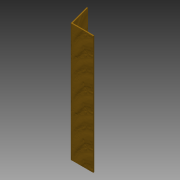
# Autodesk Inventor part: scharnierband
Saved by Autodesk Inventor 2017 (Build 210142000, 142)
## iProperties
Created: 2018-10-12
Part Number: scharnierband
Material: Brass, Soft Yellow, Welded
Document SubType Name: Modeling
Designer: ari
Density: 8.5 g/cm^3
Appearance: Weld - Brass
Author: ari
Autodesk Inventor part; units mm, degrees
ref_plane "YZ Plane" through (0, 0, 0) normal (1, 0, 0) x (0, 1, 0)
ref_plane "XZ Plane" through (0, 0, 0) normal (0, 1, 0) x (-1, 0, 0)
ref_plane "XY Plane" through (0, 0, 0) normal (0, 0, 1) x (1, 0, 0)
sketch "Sketch1" plane through (0, 0, 0) normal (0, 0, 1) x (1, 0, 0)
  line L0 (0, 0) -> (20, 0)
  line L1 (20, 0) -> (20, -1)
  line L2 (20, -1) -> (0, -1)
  line L3 (0, -1) -> (0, 0)
  line L4 (0, 0) -> (-5.1595, 19.323)
  line L5 (-5.1595, 19.323) -> (-6.1257, 19.0651)
  line L6 (-6.1257, 19.0651) -> (-0.9662, -0.258)
  line L7 (-0.9662, -0.258) -> (0, 0)
  circle A0 centre (-0.384, -0.5) radius 0.6304
  dimension "d0" = 20
  dimension "d1" = 1
  dimension "d2" = 104.95
  constraints: 16 end point, 4 parallel, 3 point on circle, 2 equal length, 2 perpendicular, 1 centre point, 1 horizontal
  measures "d0" distance of L1.end L2.end
  measures "d1" distance of L0.end L1.end
  measures "d2" angle of L4 L0
extrude "Extrusion1" add sketch "Sketch1" along normal blind 70 and the other way blind 40
body "Solid1"
